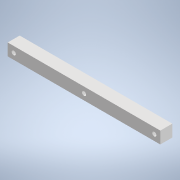
# Autodesk Inventor part: s_arm
Saved by Autodesk Inventor 2020.1 (Build 241239000, 239)
## iProperties
Created: 2019-10-17
Part Number: s_arm
Material: Generic
Document SubType Name: Modeling
Designer: jesse
Density: 1 g/cm^3
Appearance: Default
Author: jesse
Autodesk Inventor part; units mm, degrees
ref_plane "YZ Plane" through (0, 0, 0) normal (1, 0, 0) x (0, 1, 0)
ref_plane "XZ Plane" through (0, 0, 0) normal (0, 1, 0) x (-1, 0, 0)
ref_plane "XY Plane" through (0, 0, 0) normal (0, 0, 1) x (1, 0, 0)
sketch "Sketch1" plane through (0, 0, 0) normal (0, 0, 1) x (1, 0, 0)
  line L0 (0, 0) -> (58.42, 0)
  line L1 (58.42, 0) -> (58.42, 5.0161)
  line L2 (58.42, 5.0161) -> (0, 5.0161)
  line L3 (0, 5.0161) -> (0, 0)
  line L4 (29.21, 5.0161) -> (29.21, 0) construction
  circle A0 centre (29.21, 2.508) radius 1.5
  line L5 (4.4107, 5.0161) -> (4.4107, 0) construction
  line L6 (54.0093, 5.0161) -> (54.0093, 0) construction
  circle A1 centre (4.4107, 2.508) radius 1.5
  circle A2 centre (54.0093, 2.508) radius 1.5
  line L7 (4.4107, 2.508) -> (0, 2.508) construction
  line L8 (54.0093, 2.508) -> (58.42, 2.508) construction
  dimension "d0" = 58.42
  dimension "d4" = 3
  constraints: 18 end point, 7 midpoint, 4 point on line, 3 centre point, 3 perpendicular, 2 equal radius, 2 parallel, 1 collinear, 1 horizontal
  measures "d0" distance of L2.end L1.end
  measures "d4" diameter of A2
extrude "Extrusion1" add sketch "Sketch1" along normal blind 3
fillet "Fillet1" radius 2.3495 4 edges at (0, 5.0161, 1.5) (0, 0, 1.5) (58.42, 5.0161, 1.5) (58.42, 0, 1.5)
equation "\"d0\" = arm_length"
equation "\"d4\" = hole_size"
equation "\"arm_length\" = support_length"
equation "\"hole_size\" = 3"
equation "\"support_length\" = 58.42"
body "Solid1"
